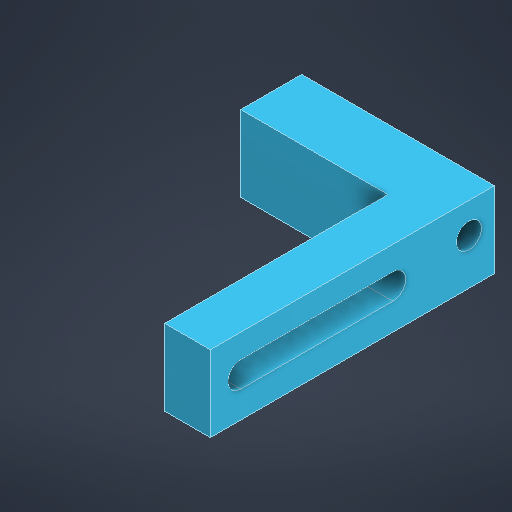
# Autodesk Inventor part: Befestigung Bremssattel
Saved by Autodesk Inventor 2026.2 (Build 302298010, 298A)
## iProperties
Created: 2026-04-15
Part Number: Befestigung Bremssattel
Material: Generisch
Document SubType Name: Modeling
Designer: pparr
Density: 1 g/cm^3
Appearance: Türkis
Author: pparr
Autodesk Inventor part; units mm, degrees
ref_plane "YZ Plane" through (0, 0, 0) normal (1, 0, 0) x (0, 1, 0)
ref_plane "XZ Plane" through (0, 0, 0) normal (0, 1, 0) x (-1, 0, 0)
ref_plane "XY Plane" through (0, 0, 0) normal (0, 0, 1) x (1, 0, 0)
sketch "Skizze1" plane through (0, 0, 0) normal (0, 1, 0) x (-1, 0, 0)
  line L0 (0, 0) -> (0, 8)
  line L1 (0, 8) -> (2, 8)
  line L2 (2, 8) -> (2, 4)
  line L3 (2, 4) -> (39, 4)
  line L4 (39, 4) -> (39, 0)
  line L5 (0, 0) -> (13.2064, 0)
  line L6 (0, 0) -> (0, -8)
  line L7 (0, -8) -> (2, -8)
  line L8 (2, -8) -> (2, -4)
  line L9 (2, -4) -> (39, -4)
  line L10 (39, -4) -> (39, 0)
  dimension "d1" = 8
  dimension "d2" = 2
  dimension "d3" = 4
  dimension "d4" = 37
  constraints: 22 end point, 4 symmetric about line, 3 perpendicular, 2 vertical, 1 horizontal
  measures "d1" distance of L0.start L0.end
  measures "d2" distance of L0.end L1.end
  measures "d3" distance of L1.end L2.end
  measures "d4" distance of L2.end L3.end
extrude "Extrusion1" add sketch "Skizze1" along normal mid plane 100
sketch "Skizze5" plane through (-39, -50, 4) normal (0, 0, 1) x (1, 0, 0)
  line L0 (0, 0) -> (0, 100) projected
  line L1 (0, 0) -> (3.5, 0)
  line L2 (3.5, 0) -> (3.5, 20)
  line L3 (3.5, 20) -> (0, 20)
  line L4 (0, 20) -> (0, 0)
  point P0 (39, 50)
  point P1 (0, 20.0912)
  dimension "d22" = 3.5
  dimension "d23" = 20
  constraints: 8 end point, 2 parallel, 1 horizontal, 1 perpendicular
  measures "d22" distance of L3.end L2.end
  measures "d23" distance of L2.end L1.end
extrude "Extrusion3" add sketch "Skizze5" along normal blind 20 and the other way blind 30
sketch "Skizze6" plane through (-39, 50, 4) normal (0, 0, 1) x (1, 0, 0)
  line L0 (0, -80) -> (0, 0) projected
  line L1 (0, 0) -> (3.5, 0)
  line L2 (3.5, 0) -> (3.5, -20)
  line L3 (3.5, -20) -> (0, -20)
  line L4 (0, -20) -> (0, 0)
  point P0 (39, -50)
  point P1 (0, -19.9088)
  point P2 (0, -20)
  dimension "d26" = 20
  dimension "d32" = 3.5
  constraints: 8 end point, 2 parallel, 1 horizontal, 1 perpendicular
  measures "d26" distance of L1.end L2.end
  measures "d32" distance between parallel lines of L0 L2
extrude "Extrusion4" add sketch "Skizze6" along normal blind 20 and the other way blind 30
sketch "Esquisse11" plane through (-35.5, 30, -4) normal (1, 0, 0) x (0, 0, -1)
  line L0 (22, 20) -> (0, 20) projected
  line L1 (22, 20) -> (22, 0) projected
  line L2 (22, -60) -> (22, -80) projected
  point P0 (-4, -30)
  point P1 (13, 7)
  point P2 (13, -67)
  dimension "d57" = 13
  dimension "d58" = 74
  dimension "d59" = 9
  dimension "d60" = 9
  measures "d57" distance from line of point (13, 7) L0
  measures "d58" distance of point (13, -67) point (13, 7)
  measures "d59" distance from line of L1 point (13, 7)
  measures "d60" distance from line of L2 point (13, -67)
hole "Perçage3" at (-35.5, 37, -17) at (-35.5, -37, -17) direction (-1, 0, 0) diameter 4.917 end through all thread size "M6x1" class "6H" standard "ISO Metric profile"
sketch "Esquisse21" plane through (-35.5, -50, 4) normal (1, 0, 0) x (0, 0, -1)
  line L0 (0, 100) -> (0, 80) projected
  line L1 (0, 20) -> (0, 80) projected
  line L2 (0, 20) -> (0, 0) projected
  line L3 (0, 100) -> (0, 0) projected
  line L4 (-36.3372, 0) -> (0, 0)
  line L5 (0, 0) -> (0, 115.7943)
  line L6 (0, 115.7943) -> (-36.3372, 115.7943)
  line L7 (-36.3372, 115.7943) -> (-36.3372, 0)
  point P0 (4, 50)
  point P1 (0, 20)
  constraints: 8 end point, 2 parallel, 1 horizontal, 1 perpendicular
extrude "Extrusion15" cut sketch "Esquisse21" along normal mid plane 9999
sketch "Esquisse28" plane through (0, 50, 0) normal (0, 1, 0) x (1, 0, 0)
  line L0 (-2, 4) -> (-35.5, 4) projected
  line L1 (-4.0336, 4) -> (2.9868, 4)
  line L2 (2.9868, 4) -> (2.9868, 11.523)
  line L3 (2.9868, 11.523) -> (-4.0336, 11.523)
  line L4 (-4.0336, 11.523) -> (-4.0336, 4)
  point P0 (0, 0)
  constraints: 8 end point, 2 parallel, 1 horizontal, 1 perpendicular, 1 point on line
extrude "Extrusion20" cut sketch "Esquisse28" against normal through all
sketch "Esquisse29" plane through (-35.5, -50, -4) normal (1, 0, 0) x (0, 0, -1)
  circle A0 centre (13, 87) radius 2.4585 projected
  line L0 (0, 80) -> (0, 100) projected
  line L1 (0, 80) -> (22, 80) projected
  line L2 (22, 100) -> (22, 80) projected
  line L3 (22, 100) -> (0, 100) projected
  circle A1 centre (13, 13) radius 2.4585 construction
  line L4 (0, 0) -> (0, 20) construction
  line L5 (22, 0) -> (0, 0) construction
  line L6 (22, 20) -> (22, 0) construction
  line L7 (0, 20) -> (22, 20) construction
  point P0 (-4, 50)
extrude "Extrusion21" add sketch "Esquisse29" along normal up to surface (35.5 mm away)
sketch "Esquisse30" plane through (0, -50, -4) normal (0, 0, -1) x (-1, 0, 0)
  line L0 (39, 80) -> (0, 80) projected
  line L1 (35.5, 0) -> (0, 0) projected
  line L2 (0, 80) -> (10, 80)
  line L3 (10, 80) -> (10, 0)
  line L4 (10, 0) -> (0, 0)
  line L5 (0, 0) -> (0, 80)
  point P0 (0, 0)
  dimension "d128" = 10
  constraints: 8 end point, 2 parallel, 1 horizontal, 1 perpendicular, 1 point on line
  measures "d128" distance between parallel lines of L5 L3
extrude "Extrusion22" add sketch "Esquisse30" along normal up to surface (22 mm away)
sketch "Esquisse31" plane through (-35.5, -30, -4) normal (0, 0, -1) x (-1, 0, 0)
  line L0 (8.9947, 60) -> (-25.5, 60)
  line L1 (-25.5, 60) -> (-25.5, -26.2912)
  line L2 (-25.5, -26.2912) -> (8.9947, -26.2912)
  line L3 (8.9947, -26.2912) -> (8.9947, 60)
  point P0 (-35.5, 30)
  constraints: 8 end point, 2 parallel, 1 horizontal, 1 perpendicular
extrude "Extrusion23" cut sketch "Esquisse31" along normal blind 100 and the other way blind 100
sketch "Esquisse32" plane through (-39, 50, -26) normal (0, 0, -1) x (-1, 0, 0)
  line L0 (-24.4847, -70) -> (-46.2931, -70)
  line L1 (-46.2931, -70) -> (-46.2931, -103.0341)
  line L2 (-46.2931, -103.0341) -> (-24.4847, -103.0341)
  line L3 (-24.4847, -103.0341) -> (-24.4847, -70)
  line L4 (-29, -100) -> (-39, -100) projected
  point P0 (-39, -50)
  dimension "d137" = 30
  constraints: 8 end point, 2 parallel, 1 horizontal, 1 perpendicular
  measures "d137" distance between parallel lines of L0 L4
extrude "Extrusion24" cut sketch "Esquisse32" against normal through all
sketch "Esquisse33" plane through (0, 50, 0) normal (0, 1, 0) x (1, 0, 0)
  line L0 (0, -4) -> (0, 26) projected
  line L1 (-39, 26) -> (-39, -4) projected
  line L2 (0, -4) -> (-39, -4)
  line L3 (-39, -4) -> (-39, 11)
  line L4 (-39, 11) -> (0, 11)
  line L5 (0, 11) -> (0, -4)
  point P0 (0, 0)
  point P1 (-39, -4)
  constraints: 8 end point, 2 parallel, 1 horizontal, 1 midpoint, 1 perpendicular
extrude "Extrusion25" cut sketch "Esquisse33" against normal through all
sketch "Esquisse34" plane through (-10, -20, -26) normal (-1, 0, 0) x (0, 0, 1)
  line L0 (7.7873, 42) -> (7.7873, 12) construction
  line L1 (5.2873, 42) -> (5.2873, 12)
  line L2 (10.2873, 12) -> (10.2873, 42)
  arc A0 (10.2873, 42) -> (5.2873, 42) centre (7.7873, 42) ccw
  arc A1 (5.2873, 12) -> (10.2873, 12) centre (7.7873, 12) ccw
  line L3 (0, 0) -> (15, 0) projected
  line L4 (0, 50) -> (15, 50) projected
  point P0 (26, 20)
  point P1 (7.7873, 27)
  dimension "d141" = 8
  dimension "d142" = 5
  dimension "d151" = 30
  constraints: 8 end point, 4 point on circle, 4 tangent, 2 centre point, 1 midpoint, 1 parallel, 1 vertical
  measures "d141" distance from line of L4 L0.start
  measures "d142" distance between parallel lines of L2 L1
  measures "d151" distance of L0.end L0.start
extrude "Extrusion26" cut sketch "Esquisse34" against normal through all
sketch "Esquisse35" plane through (0, 50, 0) normal (0, 1, 0) x (1, 0, 0)
  line L0 (-1, 5.3347) -> (8.2352, 5.3347)
  line L1 (8.2352, 5.3347) -> (8.2352, 39.622)
  line L2 (8.2352, 39.622) -> (-1, 39.622)
  line L3 (-1, 39.622) -> (-1, 5.3347)
  line L4 (0, 11) -> (0, 26) projected
  point P0 (0, 0)
  dimension "d145" = 1
  constraints: 8 end point, 2 parallel, 1 horizontal, 1 perpendicular
  measures "d145" distance between parallel lines of L4 L3
extrude "Extrusion27" cut sketch "Esquisse35" against normal through all
sketch "Esquisse36" plane through (-39, 50, -26) normal (0, 0, -1) x (-1, 0, 0)
  line L0 (7.4978, 8.0322) -> (-50.8948, 8.0322)
  line L1 (-50.8948, 8.0322) -> (-50.8948, -8)
  line L2 (-50.8948, -8) -> (7.4978, -8)
  line L3 (7.4978, -8) -> (7.4978, 8.0322)
  line L4 (0, 0) -> (-38, 0) projected
  point P0 (-39, -50)
  dimension "d148" = 8
  constraints: 8 end point, 2 parallel, 1 horizontal, 1 perpendicular
  measures "d148" distance between parallel lines of L2 L4
extrude "Extrusion28" cut sketch "Esquisse36" against normal through all
sketch "Esquisse37" plane through (-39, 50, -26) normal (0, 0, -1) x (-1, 0, 0)
  line L0 (-23.4802, -64) -> (-55.2745, -64)
  line L1 (-55.2745, -64) -> (-55.2745, -79.7659)
  line L2 (-55.2745, -79.7659) -> (-23.4802, -79.7659)
  line L3 (-23.4802, -79.7659) -> (-23.4802, -64)
  line L4 (-38, -70) -> (-29, -70) projected
  point P0 (-39, -50)
  dimension "d152" = 6
  constraints: 8 end point, 2 parallel, 1 horizontal, 1 perpendicular
  measures "d152" distance between parallel lines of L0 L4
extrude "Extrusion29" cut sketch "Esquisse37" against normal through all
